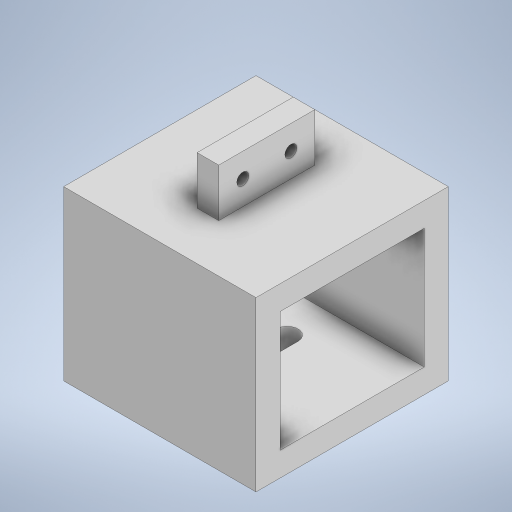
# Autodesk Inventor part: OV-PAM_slot
Saved by Autodesk Inventor 2024 (Build 280153000, 153)
## iProperties
Created: 2023-07-06
Part Number: OV-PAM_slot
Material: 일반
Document SubType Name: Modeling
Designer: jsw
Density: 1 g/cm^3
Appearance: 기본값
Author: jsw
Autodesk Inventor part; units mm, degrees
ref_plane "YZ Plane" through (0, 0, 0) normal (1, 0, 0) x (0, 1, 0)
ref_plane "XZ Plane" through (0, 0, 0) normal (0, 1, 0) x (-1, 0, 0)
ref_plane "XY Plane" through (0, 0, 0) normal (0, 0, 1) x (1, 0, 0)
sketch "스케치1" plane through (0, 0, 0) normal (0, 1, 0) x (-1, 0, 0)
  line L0 (2.25, -10) -> (-2.25, -10)
  line L1 (-2.25, -10) -> (-2.25, 10)
  line L2 (-2.25, 10) -> (2.25, 10)
  line L3 (2.25, 10) -> (2.25, -10)
  line L4 (2.25, -10) -> (-2.25, 10) construction
  line L5 (-2.25, -10) -> (2.25, 10) construction
  point P0 (0, 0)
  dimension "d0" = 4.5
  dimension "d1" = 20
  constraints: 12 end point, 2 midpoint, 2 parallel, 1 horizontal, 1 perpendicular
  measures "d0" distance of L1.end L2.end
  measures "d1" distance of L0.end L1.end
extrude "돌출1" add sketch "스케치1" along normal blind 10
sketch "스케치2" plane through (2.25, 0, 10) normal (1, 0, 0) x (0, 0, -1)
  circle A0 centre (5, 5) radius 1.25
  circle A1 centre (15, 5) radius 1.25
  line L0 (0, 0) -> (0, 10) projected
  line L1 (0, 0) -> (20, 0) projected
  point P0 (10, 0)
  point P1 (0, 5)
  dimension "d4" = 2.5
  dimension "d5" = 2.5
  dimension "d6" = 10
  dimension "d7" = 5
  dimension "d8" = 5
  constraints: 2 centre point, 1 horizontal alignment, 1 midpoint
  measures "d4" diameter of A0
  measures "d5" diameter of A1
  measures "d6" distance of A0.centre A1.centre
  measures "d7" distance of point (0, 5) A0.centre
  measures "d8" distance from line of L1 A0.centre
extrude "돌출2" cut sketch "스케치2" against normal blind 10
sketch "스케치3" plane through (0, 0, 0) normal (0, -1, 0) x (1, 0, 0)
  line L0 (-20, -20) -> (20, -20)
  line L1 (20, -20) -> (20, 20)
  line L2 (20, 20) -> (-20, 20)
  line L3 (-20, 20) -> (-20, -20)
  line L4 (-20, -20) -> (20, 20) construction
  line L5 (20, -20) -> (-20, 20) construction
  point P0 (0, 0)
  dimension "d11" = 40
  dimension "d12" = 40
  constraints: 12 end point, 2 midpoint, 2 parallel, 1 horizontal, 1 perpendicular
  measures "d11" distance of L2.end L1.end
  measures "d12" distance of L0.end L1.end
extrude "돌출3" add sketch "스케치3" along normal blind 35
shell "쉘1" thickness 5 removed faces 2 at (20, -11.6667, -6.6667) at (-20, -11.6667, 6.6667)
sketch "스케치5" plane through (0, -35, 0) normal (0, -1, 0) x (1, 0, 0)
  line L0 (0, -6.5) -> (0, 6.5) construction
  line L1 (-2.25, -6.5) -> (-2.25, 6.5)
  line L2 (2.25, 6.5) -> (2.25, -6.5)
  arc A0 (-2.25, -6.5) -> (2.25, -6.5) centre (0, -6.5) ccw
  arc A1 (2.25, 6.5) -> (-2.25, 6.5) centre (0, 6.5) ccw
  point P0 (0, 0)
  point P1 (0, 0)
  dimension "d16" = 4.5
  dimension "d17" = 13
  constraints: 8 end point, 4 point on circle, 4 tangent, 2 centre point, 1 coincident, 1 midpoint, 1 parallel, 1 vertical
  measures "d16" distance between parallel lines of L1 L2
  measures "d17" distance of L0.start L0.end
extrude "돌출4" cut sketch "스케치5" against normal up to surface (5 mm away)
